Autodesk Fusion 360 part; units mm, degrees
(part 2 of 6)
  line L897 (212.8261, -84.2499) -> (212.026, -84.2499)
  line L898 (212.026, -84.2499) -> (212.026, -78.3011)
  line L899 (212.026, -78.3011) -> (212.8261, -78.3011)
  line L900 (212.8261, -78.3011) -> (212.8261, -75.3509)
  line L901 (212.8261, -75.3509) -> (212.026, -75.3509)
  line L902 (212.026, -75.3509) -> (212.026, -74.3511)
  line L903 (212.026, -74.3511) -> (198.1761, -74.3511)
  line L904 (217.2261, -74.3511) -> (217.2261, -75.3509)
  line L905 (217.2261, -75.3509) -> (216.426, -75.3509)
  line L906 (216.426, -75.3509) -> (216.426, -78.3011)
  line L907 (216.426, -78.3011) -> (217.2261, -78.3011)
  line L908 (217.2261, -78.3011) -> (217.2261, -84.2499)
  line L909 (217.2261, -84.2499) -> (216.426, -84.2499)
  line L910 (216.426, -84.2499) -> (216.426, -87.2001)
  line L911 (216.426, -87.2001) -> (217.2261, -87.2001)
  line L912 (217.2261, -87.2001) -> (217.2261, -88.1999)
  line L913 (217.2261, -88.1999) -> (231.076, -88.1999)
  line L914 (231.076, -88.1999) -> (231.076, -87.2001)
  line L915 (231.076, -87.2001) -> (231.8761, -87.2001)
  line L916 (231.8761, -87.2001) -> (231.8761, -84.2499)
  line L917 (231.8761, -84.2499) -> (231.076, -84.2499)
  line L918 (231.076, -84.2499) -> (231.076, -78.3011)
  line L919 (231.076, -78.3011) -> (231.8761, -78.3011)
  line L920 (231.8761, -78.3011) -> (231.8761, -75.3509)
  line L921 (231.8761, -75.3509) -> (231.076, -75.3509)
  line L922 (231.076, -75.3509) -> (231.076, -74.3511)
  line L923 (231.076, -74.3511) -> (217.2261, -74.3511)
  line L924 (236.2761, -74.3511) -> (236.2761, -75.3509)
  line L925 (236.2761, -75.3509) -> (235.476, -75.3509)
  line L926 (235.476, -75.3509) -> (235.476, -78.3011)
  line L927 (235.476, -78.3011) -> (236.2761, -78.3011)
  line L928 (236.2761, -78.3011) -> (236.2761, -84.2499)
  line L929 (236.2761, -84.2499) -> (235.476, -84.2499)
  line L930 (235.476, -84.2499) -> (235.476, -87.2001)
  line L931 (235.476, -87.2001) -> (236.2761, -87.2001)
  line L932 (236.2761, -87.2001) -> (236.2761, -88.1999)
  line L933 (236.2761, -88.1999) -> (250.126, -88.1999)
  line L934 (250.126, -88.1999) -> (250.126, -87.2001)
  line L935 (250.126, -87.2001) -> (250.9261, -87.2001)
  line L936 (250.9261, -87.2001) -> (250.9261, -84.2499)
  line L937 (250.9261, -84.2499) -> (250.126, -84.2499)
  line L938 (250.126, -84.2499) -> (250.126, -78.3011)
  line L939 (250.126, -78.3011) -> (250.9261, -78.3011)
  line L940 (250.9261, -78.3011) -> (250.9261, -75.3509)
  line L941 (250.9261, -75.3509) -> (250.126, -75.3509)
  line L942 (250.126, -75.3509) -> (250.126, -74.3511)
  line L943 (250.126, -74.3511) -> (236.2761, -74.3511)
  line L944 (307.7131, -74.3511) -> (307.7131, -75.3509)
  line L945 (307.7131, -75.3509) -> (306.914, -75.3509)
  line L946 (306.914, -75.3509) -> (306.914, -78.3011)
  line L947 (306.914, -78.3011) -> (307.7131, -78.3011)
  line L948 (307.7131, -78.3011) -> (307.7131, -84.2499)
  line L949 (307.7131, -84.2499) -> (306.914, -84.2499)
  line L950 (306.914, -84.2499) -> (306.914, -87.2001)
  line L951 (306.914, -87.2001) -> (307.7131, -87.2001)
  line L952 (307.7131, -87.2001) -> (307.7131, -88.1999)
  line L953 (307.7131, -88.1999) -> (321.564, -88.1999)
  line L954 (321.564, -88.1999) -> (321.564, -87.2001)
  line L955 (321.564, -87.2001) -> (322.363, -87.2001)
  line L956 (322.363, -87.2001) -> (322.363, -84.2499)
  line L957 (322.363, -84.2499) -> (321.564, -84.2499)
  line L958 (321.564, -84.2499) -> (321.564, -78.3011)
  line L959 (321.564, -78.3011) -> (322.363, -78.3011)
  line L960 (322.363, -78.3011) -> (322.363, -75.3509)
  line L961 (322.363, -75.3509) -> (321.564, -75.3509)
  line L962 (321.564, -75.3509) -> (321.564, -74.3511)
  line L963 (321.564, -74.3511) -> (307.7131, -74.3511)
  line L964 (17.201, -55.3011) -> (17.201, -56.301)
  line L965 (17.201, -56.301) -> (16.401, -56.301)
  line L966 (16.401, -56.301) -> (16.401, -59.25)
  line L967 (16.401, -59.25) -> (17.201, -59.25)
  line L968 (17.201, -59.25) -> (17.201, -65.1999)
  line L969 (17.201, -65.1999) -> (16.401, -65.1999)
  line L970 (16.401, -65.1999) -> (16.401, -68.1501)
  line L971 (16.401, -68.1501) -> (17.201, -68.1501)
  line L972 (17.201, -68.1501) -> (17.201, -69.1499)
  line L973 (17.201, -69.1499) -> (31.051, -69.1499)
  line L974 (31.051, -69.1499) -> (31.051, -68.1501)
  line L975 (31.051, -68.1501) -> (31.8511, -68.1501)
  line L976 (31.8511, -68.1501) -> (31.8511, -65.1999)
  line L977 (31.8511, -65.1999) -> (31.051, -65.1999)
  line L978 (31.051, -65.1999) -> (31.051, -59.25)
  line L979 (31.051, -59.25) -> (31.8511, -59.25)
  line L980 (31.8511, -59.25) -> (31.8511, -56.301)
  line L981 (31.8511, -56.301) -> (31.051, -56.301)
  line L982 (31.051, -56.301) -> (31.051, -55.3011)
  line L983 (31.051, -55.3011) -> (17.201, -55.3011)
  line L984 (41.0131, -55.3011) -> (41.0131, -56.301)
  line L985 (41.0131, -56.301) -> (40.213, -56.301)
  line L986 (40.213, -56.301) -> (40.213, -59.25)
  line L987 (40.213, -59.25) -> (41.0131, -59.25)
  line L988 (41.0131, -59.25) -> (41.0131, -65.1999)
  line L989 (41.0131, -65.1999) -> (40.213, -65.1999)
  line L990 (40.213, -65.1999) -> (40.213, -68.1501)
  line L991 (40.213, -68.1501) -> (41.0131, -68.1501)
  line L992 (41.0131, -68.1501) -> (41.0131, -69.1499)
  line L993 (41.0131, -69.1499) -> (54.8629, -69.1499)
  line L994 (54.8629, -69.1499) -> (54.8629, -68.1501)
  line L995 (54.8629, -68.1501) -> (55.663, -68.1501)
  line L996 (55.663, -68.1501) -> (55.663, -65.1999)
  line L997 (55.663, -65.1999) -> (54.8629, -65.1999)
  line L998 (54.8629, -65.1999) -> (54.8629, -59.25)
  line L999 (54.8629, -59.25) -> (55.663, -59.25)
  line L1000 (55.663, -59.25) -> (55.663, -56.301)
  line L1001 (55.663, -56.301) -> (54.8629, -56.301)
  line L1002 (54.8629, -56.301) -> (54.8629, -55.3011)
  line L1003 (54.8629, -55.3011) -> (41.0131, -55.3011)
  line L1004 (60.0631, -55.3011) -> (60.0631, -56.301)
  line L1005 (60.0631, -56.301) -> (59.263, -56.301)
  line L1006 (59.263, -56.301) -> (59.263, -59.25)
  line L1007 (59.263, -59.25) -> (60.0631, -59.25)
  line L1008 (60.0631, -59.25) -> (60.0631, -65.1999)
  line L1009 (60.0631, -65.1999) -> (59.263, -65.1999)
  line L1010 (59.263, -65.1999) -> (59.263, -68.1501)
  line L1011 (59.263, -68.1501) -> (60.0631, -68.1501)
  line L1012 (60.0631, -68.1501) -> (60.0631, -69.1499)
  line L1013 (60.0631, -69.1499) -> (73.9129, -69.1499)
  line L1014 (73.9129, -69.1499) -> (73.9129, -68.1501)
  line L1015 (73.9129, -68.1501) -> (74.713, -68.1501)
  line L1016 (74.713, -68.1501) -> (74.713, -65.1999)
  line L1017 (74.713, -65.1999) -> (73.9129, -65.1999)
  line L1018 (73.9129, -65.1999) -> (73.9129, -59.25)
  line L1019 (73.9129, -59.25) -> (74.713, -59.25)
  line L1020 (74.713, -59.25) -> (74.713, -56.301)
  line L1021 (74.713, -56.301) -> (73.9129, -56.301)
  line L1022 (73.9129, -56.301) -> (73.9129, -55.3011)
  line L1023 (73.9129, -55.3011) -> (60.0631, -55.3011)
  line L1024 (79.1131, -55.3011) -> (79.1131, -56.301)
  line L1025 (79.1131, -56.301) -> (78.313, -56.301)
  line L1026 (78.313, -56.301) -> (78.313, -59.25)
  line L1027 (78.313, -59.25) -> (79.1131, -59.25)
  line L1028 (79.1131, -59.25) -> (79.1131, -65.1999)
  line L1029 (79.1131, -65.1999) -> (78.313, -65.1999)
  line L1030 (78.313, -65.1999) -> (78.313, -68.1501)
  line L1031 (78.313, -68.1501) -> (79.1131, -68.1501)
  line L1032 (79.1131, -68.1501) -> (79.1131, -69.1499)
  line L1033 (79.1131, -69.1499) -> (92.9629, -69.1499)
  line L1034 (92.9629, -69.1499) -> (92.9629, -68.1501)
  line L1035 (92.9629, -68.1501) -> (93.763, -68.1501)
  line L1036 (93.763, -68.1501) -> (93.763, -65.1999)
  line L1037 (93.763, -65.1999) -> (92.9629, -65.1999)
  line L1038 (92.9629, -65.1999) -> (92.9629, -59.25)
  line L1039 (92.9629, -59.25) -> (93.763, -59.25)
  line L1040 (93.763, -59.25) -> (93.763, -56.301)
  line L1041 (93.763, -56.301) -> (92.9629, -56.301)
  line L1042 (92.9629, -56.301) -> (92.9629, -55.3011)
  line L1043 (92.9629, -55.3011) -> (79.1131, -55.3011)
  line L1044 (98.1631, -55.3011) -> (98.1631, -56.301)
  line L1045 (98.1631, -56.301) -> (97.363, -56.301)
  line L1046 (97.363, -56.301) -> (97.363, -59.25)
  line L1047 (97.363, -59.25) -> (98.1631, -59.25)
  line L1048 (98.1631, -59.25) -> (98.1631, -65.1999)
  line L1049 (98.1631, -65.1999) -> (97.363, -65.1999)
  line L1050 (97.363, -65.1999) -> (97.363, -68.1501)
  line L1051 (97.363, -68.1501) -> (98.1631, -68.1501)
  line L1052 (98.1631, -68.1501) -> (98.1631, -69.1499)
  line L1053 (98.1631, -69.1499) -> (112.0129, -69.1499)
  line L1054 (112.0129, -69.1499) -> (112.0129, -68.1501)
  line L1055 (112.0129, -68.1501) -> (112.813, -68.1501)
  line L1056 (112.813, -68.1501) -> (112.813, -65.1999)
  line L1057 (112.813, -65.1999) -> (112.0129, -65.1999)
  line L1058 (112.0129, -65.1999) -> (112.0129, -59.25)
  line L1059 (112.0129, -59.25) -> (112.813, -59.25)
  line L1060 (112.813, -59.25) -> (112.813, -56.301)
  line L1061 (112.813, -56.301) -> (112.0129, -56.301)
  line L1062 (112.0129, -56.301) -> (112.0129, -55.3011)
  line L1063 (112.0129, -55.3011) -> (98.1631, -55.3011)
  line L1064 (117.2131, -55.3011) -> (117.2131, -56.301)
  line L1065 (117.2131, -56.301) -> (116.413, -56.301)
  line L1066 (116.413, -56.301) -> (116.413, -59.25)
  line L1067 (116.413, -59.25) -> (117.2131, -59.25)
  line L1068 (117.2131, -59.25) -> (117.2131, -65.1999)
  line L1069 (117.2131, -65.1999) -> (116.413, -65.1999)
  line L1070 (116.413, -65.1999) -> (116.413, -68.1501)
  line L1071 (116.413, -68.1501) -> (117.2131, -68.1501)
  line L1072 (117.2131, -68.1501) -> (117.2131, -69.1499)
  line L1073 (117.2131, -69.1499) -> (131.0629, -69.1499)
  line L1074 (131.0629, -69.1499) -> (131.0629, -68.1501)
  line L1075 (131.0629, -68.1501) -> (131.863, -68.1501)
  line L1076 (131.863, -68.1501) -> (131.863, -65.1999)
  line L1077 (131.863, -65.1999) -> (131.0629, -65.1999)
  line L1078 (131.0629, -65.1999) -> (131.0629, -59.25)
  line L1079 (131.0629, -59.25) -> (131.863, -59.25)
  line L1080 (131.863, -59.25) -> (131.863, -56.301)
  line L1081 (131.863, -56.301) -> (131.0629, -56.301)
  line L1082 (131.0629, -56.301) -> (131.0629, -55.3011)
  line L1083 (131.0629, -55.3011) -> (117.2131, -55.3011)
  line L1084 (136.2631, -55.3011) -> (136.2631, -56.301)
  line L1085 (136.2631, -56.301) -> (135.463, -56.301)
  line L1086 (135.463, -56.301) -> (135.463, -59.25)
  line L1087 (135.463, -59.25) -> (136.2631, -59.25)
  line L1088 (136.2631, -59.25) -> (136.2631, -65.1999)
  line L1089 (136.2631, -65.1999) -> (135.463, -65.1999)
  line L1090 (135.463, -65.1999) -> (135.463, -68.1501)
  line L1091 (135.463, -68.1501) -> (136.2631, -68.1501)
  line L1092 (136.2631, -68.1501) -> (136.2631, -69.1499)
  line L1093 (136.2631, -69.1499) -> (150.1129, -69.1499)
  line L1094 (150.1129, -69.1499) -> (150.1129, -68.1501)
  line L1095 (150.1129, -68.1501) -> (150.913, -68.1501)
  line L1096 (150.913, -68.1501) -> (150.913, -65.1999)
  line L1097 (150.913, -65.1999) -> (150.1129, -65.1999)
  line L1098 (150.1129, -65.1999) -> (150.1129, -59.25)
  line L1099 (150.1129, -59.25) -> (150.913, -59.25)
  line L1100 (150.913, -59.25) -> (150.913, -56.301)
  line L1101 (150.913, -56.301) -> (150.1129, -56.301)
  line L1102 (150.1129, -56.301) -> (150.1129, -55.3011)
  line L1103 (150.1129, -55.3011) -> (136.2631, -55.3011)
  line L1104 (155.3131, -55.3011) -> (155.3131, -56.301)
  line L1105 (155.3131, -56.301) -> (154.513, -56.301)
  line L1106 (154.513, -56.301) -> (154.513, -59.25)
  line L1107 (154.513, -59.25) -> (155.3131, -59.25)
  line L1108 (155.3131, -59.25) -> (155.3131, -65.1999)
  line L1109 (155.3131, -65.1999) -> (154.513, -65.1999)
  line L1110 (154.513, -65.1999) -> (154.513, -68.1501)
  line L1111 (154.513, -68.1501) -> (155.3131, -68.1501)
  line L1112 (155.3131, -68.1501) -> (155.3131, -69.1499)
  line L1113 (155.3131, -69.1499) -> (169.1629, -69.1499)
  line L1114 (169.1629, -69.1499) -> (169.1629, -68.1501)
  line L1115 (169.1629, -68.1501) -> (169.963, -68.1501)
  line L1116 (169.963, -68.1501) -> (169.963, -65.1999)
  line L1117 (169.963, -65.1999) -> (169.1629, -65.1999)
  line L1118 (169.1629, -65.1999) -> (169.1629, -59.25)
  line L1119 (169.1629, -59.25) -> (169.963, -59.25)
  line L1120 (169.963, -59.25) -> (169.963, -56.301)
  line L1121 (169.963, -56.301) -> (169.1629, -56.301)
  line L1122 (169.1629, -56.301) -> (169.1629, -55.3011)
  line L1123 (169.1629, -55.3011) -> (155.3131, -55.3011)
  line L1124 (174.3631, -55.3011) -> (174.3631, -56.301)
  line L1125 (174.3631, -56.301) -> (173.563, -56.301)
  line L1126 (173.563, -56.301) -> (173.563, -59.25)
  line L1127 (173.563, -59.25) -> (174.3631, -59.25)
  line L1128 (174.3631, -59.25) -> (174.3631, -65.1999)
  line L1129 (174.3631, -65.1999) -> (173.563, -65.1999)
  line L1130 (173.563, -65.1999) -> (173.563, -68.1501)
  line L1131 (173.563, -68.1501) -> (174.3631, -68.1501)
  line L1132 (174.3631, -68.1501) -> (174.3631, -69.1499)
  line L1133 (174.3631, -69.1499) -> (188.2129, -69.1499)
  line L1134 (188.2129, -69.1499) -> (188.2129, -68.1501)
  line L1135 (188.2129, -68.1501) -> (189.013, -68.1501)
  line L1136 (189.013, -68.1501) -> (189.013, -65.1999)
  line L1137 (189.013, -65.1999) -> (188.2129, -65.1999)
  line L1138 (188.2129, -65.1999) -> (188.2129, -59.25)
  line L1139 (188.2129, -59.25) -> (189.013, -59.25)
  line L1140 (189.013, -59.25) -> (189.013, -56.301)
  line L1141 (189.013, -56.301) -> (188.2129, -56.301)
  line L1142 (188.2129, -56.301) -> (188.2129, -55.3011)
  line L1143 (188.2129, -55.3011) -> (174.3631, -55.3011)
  line L1144 (193.4131, -55.3011) -> (193.4131, -56.301)
  line L1145 (193.4131, -56.301) -> (192.613, -56.301)
  line L1146 (192.613, -56.301) -> (192.613, -59.25)
  line L1147 (192.613, -59.25) -> (193.4131, -59.25)
  line L1148 (193.4131, -59.25) -> (193.4131, -65.1999)
  line L1149 (193.4131, -65.1999) -> (192.613, -65.1999)
  line L1150 (192.613, -65.1999) -> (192.613, -68.1501)
  line L1151 (192.613, -68.1501) -> (193.4131, -68.1501)
  line L1152 (193.4131, -68.1501) -> (193.4131, -69.1499)
  line L1153 (193.4131, -69.1499) -> (207.2629, -69.1499)
  line L1154 (207.2629, -69.1499) -> (207.2629, -68.1501)
  line L1155 (207.2629, -68.1501) -> (208.063, -68.1501)
  line L1156 (208.063, -68.1501) -> (208.063, -65.1999)
  line L1157 (208.063, -65.1999) -> (207.2629, -65.1999)
  line L1158 (207.2629, -65.1999) -> (207.2629, -59.25)
  line L1159 (207.2629, -59.25) -> (208.063, -59.25)
  line L1160 (208.063, -59.25) -> (208.063, -56.301)
  line L1161 (208.063, -56.301) -> (207.2629, -56.301)
  line L1162 (207.2629, -56.301) -> (207.2629, -55.3011)
  line L1163 (207.2629, -55.3011) -> (193.4131, -55.3011)
  line L1164 (212.4631, -55.3011) -> (212.4631, -56.301)
  line L1165 (212.4631, -56.301) -> (211.663, -56.301)
  line L1166 (211.663, -56.301) -> (211.663, -59.25)
  line L1167 (211.663, -59.25) -> (212.4631, -59.25)
  line L1168 (212.4631, -59.25) -> (212.4631, -65.1999)
  line L1169 (212.4631, -65.1999) -> (211.663, -65.1999)
  line L1170 (211.663, -65.1999) -> (211.663, -68.1501)
  line L1171 (211.663, -68.1501) -> (212.4631, -68.1501)
  line L1172 (212.4631, -68.1501) -> (212.4631, -69.1499)
  line L1173 (212.4631, -69.1499) -> (226.3129, -69.1499)
  line L1174 (226.3129, -69.1499) -> (226.3129, -68.1501)
  line L1175 (226.3129, -68.1501) -> (227.113, -68.1501)
  line L1176 (227.113, -68.1501) -> (227.113, -65.1999)
  line L1177 (227.113, -65.1999) -> (226.3129, -65.1999)
  line L1178 (226.3129, -65.1999) -> (226.3129, -59.25)
  line L1179 (226.3129, -59.25) -> (227.113, -59.25)
  line L1180 (227.113, -59.25) -> (227.113, -56.301)
  line L1181 (227.113, -56.301) -> (226.3129, -56.301)
  line L1182 (226.3129, -56.301) -> (226.3129, -55.3011)
  line L1183 (226.3129, -55.3011) -> (212.4631, -55.3011)
  line L1184 (231.5131, -55.3011) -> (231.5131, -56.301)
  line L1185 (231.5131, -56.301) -> (230.713, -56.301)
  line L1186 (230.713, -56.301) -> (230.713, -59.25)
  line L1187 (230.713, -59.25) -> (231.5131, -59.25)
  line L1188 (231.5131, -59.25) -> (231.5131, -65.1999)
  line L1189 (231.5131, -65.1999) -> (230.713, -65.1999)
  line L1190 (230.713, -65.1999) -> (230.713, -68.1501)
  line L1191 (230.713, -68.1501) -> (231.5131, -68.1501)
  line L1192 (231.5131, -68.1501) -> (231.5131, -69.1499)
  line L1193 (231.5131, -69.1499) -> (245.3629, -69.1499)
  line L1194 (245.3629, -69.1499) -> (245.3629, -68.1501)
  line L1195 (245.3629, -68.1501) -> (246.163, -68.1501)
  line L1196 (246.163, -68.1501) -> (246.163, -65.1999)
  line L1197 (246.163, -65.1999) -> (245.3629, -65.1999)
  line L1198 (245.3629, -65.1999) -> (245.3629, -59.25)
  line L1199 (245.3629, -59.25) -> (246.163, -59.25)
  line L1200 (246.163, -59.25) -> (246.163, -56.301)
  line L1201 (246.163, -56.301) -> (245.3629, -56.301)
  line L1202 (245.3629, -56.301) -> (245.3629, -55.3011)
  line L1203 (245.3629, -55.3011) -> (231.5131, -55.3011)
  line L1204 (250.5631, -55.3011) -> (250.5631, -56.301)
  line L1205 (250.5631, -56.301) -> (249.763, -56.301)
  line L1206 (249.763, -56.301) -> (249.763, -59.25)
  line L1207 (249.763, -59.25) -> (250.5631, -59.25)
  line L1208 (250.5631, -59.25) -> (250.5631, -65.1999)
  line L1209 (250.5631, -65.1999) -> (249.763, -65.1999)
  line L1210 (249.763, -65.1999) -> (249.763, -68.1501)
  line L1211 (249.763, -68.1501) -> (250.5631, -68.1501)
  line L1212 (250.5631, -68.1501) -> (250.5631, -69.1499)
  line L1213 (250.5631, -69.1499) -> (264.4129, -69.1499)
  line L1214 (264.4129, -69.1499) -> (264.4129, -68.1501)
  line L1215 (264.4129, -68.1501) -> (265.213, -68.1501)
  line L1216 (265.213, -68.1501) -> (265.213, -65.1999)
  line L1217 (265.213, -65.1999) -> (264.4129, -65.1999)
  line L1218 (264.4129, -65.1999) -> (264.4129, -59.25)
  line L1219 (264.4129, -59.25) -> (265.213, -59.25)
  line L1220 (265.213, -59.25) -> (265.213, -56.301)
  line L1221 (265.213, -56.301) -> (264.4129, -56.301)
  line L1222 (264.4129, -56.301) -> (264.4129, -55.3011)
  line L1223 (264.4129, -55.3011) -> (250.5631, -55.3011)
  line L1224 (274.3756, -55.3011) -> (274.3756, -56.301)
  line L1225 (274.3756, -56.301) -> (273.5765, -56.301)
  line L1226 (273.5765, -56.301) -> (273.5765, -59.25)
  line L1227 (273.5765, -59.25) -> (274.3756, -59.25)
  line L1228 (274.3756, -59.25) -> (274.3756, -65.1999)
  line L1229 (274.3756, -65.1999) -> (273.5765, -65.1999)
  line L1230 (273.5765, -65.1999) -> (273.5765, -68.1501)
  line L1231 (273.5765, -68.1501) -> (274.3756, -68.1501)
  line L1232 (274.3756, -68.1501) -> (274.3756, -69.1499)
  line L1233 (274.3756, -69.1499) -> (288.2265, -69.1499)
  line L1234 (288.2265, -69.1499) -> (288.2265, -68.1501)
  line L1235 (288.2265, -68.1501) -> (289.0255, -68.1501)
  line L1236 (289.0255, -68.1501) -> (289.0255, -65.1999)
  line L1237 (289.0255, -65.1999) -> (288.2265, -65.1999)
  line L1238 (288.2265, -65.1999) -> (288.2265, -59.25)
  line L1239 (288.2265, -59.25) -> (289.0255, -59.25)
  line L1240 (289.0255, -59.25) -> (289.0255, -56.301)
  line L1241 (289.0255, -56.301) -> (288.2265, -56.301)
  line L1242 (288.2265, -56.301) -> (288.2265, -55.3011)
  line L1243 (288.2265, -55.3011) -> (274.3756, -55.3011)
  line L1244 (307.7131, -55.3011) -> (307.7131, -56.301)
  line L1245 (307.7131, -56.301) -> (306.914, -56.301)
  line L1246 (306.914, -56.301) -> (306.914, -59.25)
  line L1247 (306.914, -59.25) -> (307.7131, -59.25)
  line L1248 (307.7131, -59.25) -> (307.7131, -65.1999)
  line L1249 (307.7131, -65.1999) -> (306.914, -65.1999)
  line L1250 (306.914, -65.1999) -> (306.914, -68.1501)
  line L1251 (306.914, -68.1501) -> (307.7131, -68.1501)
  line L1252 (307.7131, -68.1501) -> (307.7131, -69.1499)
  line L1253 (307.7131, -69.1499) -> (321.564, -69.1499)
  line L1254 (321.564, -69.1499) -> (321.564, -68.1501)
  line L1255 (321.564, -68.1501) -> (322.363, -68.1501)
  line L1256 (322.363, -68.1501) -> (322.363, -65.1999)
  line L1257 (322.363, -65.1999) -> (321.564, -65.1999)
  line L1258 (321.564, -65.1999) -> (321.564, -59.25)
  line L1259 (321.564, -59.25) -> (322.363, -59.25)
  line L1260 (322.363, -59.25) -> (322.363, -56.301)
  line L1261 (322.363, -56.301) -> (321.564, -56.301)
  line L1262 (321.564, -56.301) -> (321.564, -55.3011)
  line L1263 (321.564, -55.3011) -> (307.7131, -55.3011)
  line L1264 (269.6131, -36.2511) -> (269.6131, -37.251)
  line L1265 (269.6131, -37.251) -> (268.814, -37.251)
  line L1266 (268.814, -37.251) -> (268.814, -40.2)
  line L1267 (268.814, -40.2) -> (269.6131, -40.2)
  line L1268 (269.6131, -40.2) -> (269.6131, -40.9501)
  line L1269 (269.6131, -40.9501) -> (267.9382, -40.9501)
  line L1270 (267.9382, -40.9501) -> (267.9382, -37.7211)
  line L1271 (267.9382, -37.7211) -> (266.2132, -37.7211)
  line L1272 (266.2132, -37.7211) -> (266.2132, -36.8009)
  line L1273 (266.2132, -36.8009) -> (263.063, -36.8009)
  line L1274 (263.063, -36.8009) -> (263.063, -37.7211)
  line L1275 (263.063, -37.7211) -> (261.338, -37.7211)
  line L1276 (261.338, -37.7211) -> (261.338, -40.9501)
  line L1277 (261.338, -40.9501) -> (260.513, -40.9501)
  line L1278 (260.513, -40.9501) -> (260.513, -43.5999)
  line L1279 (260.513, -43.5999) -> (261.338, -43.5999)
  line L1280 (261.338, -43.5999) -> (261.338, -49.871)
  line L1281 (261.338, -49.871) -> (263.063, -49.871)
  line L1282 (263.063, -49.871) -> (263.063, -50.85)
  line L1283 (263.063, -50.85) -> (266.2132, -50.85)
  line L1284 (266.2132, -50.85) -> (266.2132, -49.871)
  line L1285 (266.2132, -49.871) -> (267.9382, -49.871)
  line L1286 (267.9382, -49.871) -> (267.9382, -45.4009)
  line L1287 (267.9382, -45.4009) -> (269.6131, -45.4009)
  line L1288 (269.6131, -45.4009) -> (269.6131, -46.151)
  line L1289 (269.6131, -46.151) -> (268.814, -46.151)
  line L1290 (268.814, -46.151) -> (268.814, -49.1001)
  line L1291 (268.814, -49.1001) -> (269.6131, -49.1001)
  line L1292 (269.6131, -49.1001) -> (269.6131, -50.0999)
  line L1293 (269.6131, -50.0999) -> (283.464, -50.0999)
  line L1294 (283.464, -50.0999) -> (283.464, -49.1001)
  line L1295 (283.464, -49.1001) -> (284.263, -49.1001)
  line L1296 (284.263, -49.1001) -> (284.263, -46.151)
  line L1297 (284.263, -46.151) -> (283.464, -46.151)
  line L1298 (283.464, -46.151) -> (283.464, -45.4009)
  line L1299 (283.464, -45.4009) -> (285.1388, -45.4009)
  line L1300 (285.1388, -45.4009) -> (285.1388, -49.871)
  line L1301 (285.1388, -49.871) -> (286.8639, -49.871)
  line L1302 (286.8639, -49.871) -> (286.8639, -50.85)
  line L1303 (286.8639, -50.85) -> (290.0124, -50.85)
  line L1304 (290.0124, -50.85) -> (290.0124, -49.871)
  line L1305 (290.0124, -49.871) -> (291.7375, -49.871)
  line L1306 (291.7375, -49.871) -> (291.7375, -43.5999)
  line L1307 (291.7375, -43.5999) -> (292.563, -43.5999)
  line L1308 (292.563, -43.5999) -> (292.563, -40.9501)
  line L1309 (292.563, -40.9501) -> (291.7375, -40.9501)
  line L1310 (291.7375, -40.9501) -> (291.7375, -37.7211)
  line L1311 (291.7375, -37.7211) -> (290.0124, -37.7211)
  line L1312 (290.0124, -37.7211) -> (290.0124, -36.8009)
  line L1313 (290.0124, -36.8009) -> (286.8639, -36.8009)
  line L1314 (286.8639, -36.8009) -> (286.8639, -37.7211)
  line L1315 (286.8639, -37.7211) -> (285.1388, -37.7211)
  line L1316 (285.1388, -37.7211) -> (285.1388, -40.9501)
  line L1317 (285.1388, -40.9501) -> (283.464, -40.9501)
  line L1318 (283.464, -40.9501) -> (283.464, -40.2)
  line L1319 (283.464, -40.2) -> (284.263, -40.2)
  line L1320 (284.263, -40.2) -> (284.263, -37.251)
  line L1321 (284.263, -37.251) -> (283.464, -37.251)
  line L1322 (283.464, -37.251) -> (283.464, -36.2511)
  line L1323 (283.464, -36.2511) -> (269.6131, -36.2511)
  line L1324 (12.438, -36.2511) -> (12.438, -37.251)
  line L1325 (12.438, -37.251) -> (11.638, -37.251)
  line L1326 (11.638, -37.251) -> (11.638, -40.2)
  line L1327 (11.638, -40.2) -> (12.438, -40.2)
  line L1328 (12.438, -40.2) -> (12.438, -46.151)
  line L1329 (12.438, -46.151) -> (11.638, -46.151)
  line L1330 (11.638, -46.151) -> (11.638, -49.1001)
  line L1331 (11.638, -49.1001) -> (12.438, -49.1001)
  line L1332 (12.438, -49.1001) -> (12.438, -50.0999)
  line L1333 (12.438, -50.0999) -> (26.288, -50.0999)
  line L1334 (26.288, -50.0999) -> (26.288, -49.1001)
  line L1335 (26.288, -49.1001) -> (27.088, -49.1001)
  line L1336 (27.088, -49.1001) -> (27.088, -46.151)
  line L1337 (27.088, -46.151) -> (26.288, -46.151)
  line L1338 (26.288, -46.151) -> (26.288, -40.2)
  line L1339 (26.288, -40.2) -> (27.088, -40.2)
  line L1340 (27.088, -40.2) -> (27.088, -37.251)
  line L1341 (27.088, -37.251) -> (26.288, -37.251)
  line L1342 (26.288, -37.251) -> (26.288, -36.2511)
  line L1343 (26.288, -36.2511) -> (12.438, -36.2511)
  line L1344 (31.4881, -36.2511) -> (31.4881, -37.251)
  line L1345 (31.4881, -37.251) -> (30.688, -37.251)
  line L1346 (30.688, -37.251) -> (30.688, -40.2)
  line L1347 (30.688, -40.2) -> (31.4881, -40.2)
  line L1348 (31.4881, -40.2) -> (31.4881, -46.151)
  line L1349 (31.4881, -46.151) -> (30.688, -46.151)
  line L1350 (30.688, -46.151) -> (30.688, -49.1001)
  line L1351 (30.688, -49.1001) -> (31.4881, -49.1001)
  line L1352 (31.4881, -49.1001) -> (31.4881, -50.0999)
  line L1353 (31.4881, -50.0999) -> (45.3379, -50.0999)
  line L1354 (45.3379, -50.0999) -> (45.3379, -49.1001)
  line L1355 (45.3379, -49.1001) -> (46.138, -49.1001)
  line L1356 (46.138, -49.1001) -> (46.138, -46.151)
  line L1357 (46.138, -46.151) -> (45.3379, -46.151)
  line L1358 (45.3379, -46.151) -> (45.3379, -40.2)
  line L1359 (45.3379, -40.2) -> (46.138, -40.2)
  line L1360 (46.138, -40.2) -> (46.138, -37.251)
  line L1361 (46.138, -37.251) -> (45.3379, -37.251)
  line L1362 (45.3379, -37.251) -> (45.3379, -36.2511)
  line L1363 (45.3379, -36.2511) -> (31.4881, -36.2511)
  line L1364 (50.5381, -36.2511) -> (50.5381, -37.251)
  line L1365 (50.5381, -37.251) -> (49.738, -37.251)
  line L1366 (49.738, -37.251) -> (49.738, -40.2)
  line L1367 (49.738, -40.2) -> (50.5381, -40.2)
  line L1368 (50.5381, -40.2) -> (50.5381, -46.151)
  line L1369 (50.5381, -46.151) -> (49.738, -46.151)
  line L1370 (49.738, -46.151) -> (49.738, -49.1001)
  line L1371 (49.738, -49.1001) -> (50.5381, -49.1001)
  line L1372 (50.5381, -49.1001) -> (50.5381, -50.0999)
  line L1373 (50.5381, -50.0999) -> (64.3879, -50.0999)
  line L1374 (64.3879, -50.0999) -> (64.3879, -49.1001)
  line L1375 (64.3879, -49.1001) -> (65.188, -49.1001)
  line L1376 (65.188, -49.1001) -> (65.188, -46.151)
  line L1377 (65.188, -46.151) -> (64.3879, -46.151)
  line L1378 (64.3879, -46.151) -> (64.3879, -40.2)
  line L1379 (64.3879, -40.2) -> (65.188, -40.2)
  line L1380 (65.188, -40.2) -> (65.188, -37.251)
  line L1381 (65.188, -37.251) -> (64.3879, -37.251)
  line L1382 (64.3879, -37.251) -> (64.3879, -36.2511)
  line L1383 (64.3879, -36.2511) -> (50.5381, -36.2511)
  line L1384 (69.5881, -36.2511) -> (69.5881, -37.251)
  line L1385 (69.5881, -37.251) -> (68.788, -37.251)
  line L1386 (68.788, -37.251) -> (68.788, -40.2)
  line L1387 (68.788, -40.2) -> (69.5881, -40.2)
  line L1388 (69.5881, -40.2) -> (69.5881, -46.151)
  line L1389 (69.5881, -46.151) -> (68.788, -46.151)
  line L1390 (68.788, -46.151) -> (68.788, -49.1001)
  line L1391 (68.788, -49.1001) -> (69.5881, -49.1001)
  line L1392 (69.5881, -49.1001) -> (69.5881, -50.0999)
  line L1393 (69.5881, -50.0999) -> (83.4379, -50.0999)
  line L1394 (83.4379, -50.0999) -> (83.4379, -49.1001)
  line L1395 (83.4379, -49.1001) -> (84.238, -49.1001)
  line L1396 (84.238, -49.1001) -> (84.238, -46.151)
  line L1397 (84.238, -46.151) -> (83.4379, -46.151)
  line L1398 (83.4379, -46.151) -> (83.4379, -40.2)
  line L1399 (83.4379, -40.2) -> (84.238, -40.2)
  line L1400 (84.238, -40.2) -> (84.238, -37.251)
  line L1401 (84.238, -37.251) -> (83.4379, -37.251)
  line L1402 (83.4379, -37.251) -> (83.4379, -36.2511)
  line L1403 (83.4379, -36.2511) -> (69.5881, -36.2511)
  line L1404 (88.6381, -36.2511) -> (88.6381, -37.251)
  line L1405 (88.6381, -37.251) -> (87.838, -37.251)
  line L1406 (87.838, -37.251) -> (87.838, -40.2)
  line L1407 (87.838, -40.2) -> (88.6381, -40.2)
  line L1408 (88.6381, -40.2) -> (88.6381, -46.151)
  line L1409 (88.6381, -46.151) -> (87.838, -46.151)
  line L1410 (87.838, -46.151) -> (87.838, -49.1001)
  line L1411 (87.838, -49.1001) -> (88.6381, -49.1001)
  line L1412 (88.6381, -49.1001) -> (88.6381, -50.0999)
  line L1413 (88.6381, -50.0999) -> (102.4879, -50.0999)
  line L1414 (102.4879, -50.0999) -> (102.4879, -49.1001)
  line L1415 (102.4879, -49.1001) -> (103.288, -49.1001)
  line L1416 (103.288, -49.1001) -> (103.288, -46.151)
  line L1417 (103.288, -46.151) -> (102.4879, -46.151)
  line L1418 (102.4879, -46.151) -> (102.4879, -40.2)
  line L1419 (102.4879, -40.2) -> (103.288, -40.2)
  line L1420 (103.288, -40.2) -> (103.288, -37.251)
  line L1421 (103.288, -37.251) -> (102.4879, -37.251)
  line L1422 (102.4879, -37.251) -> (102.4879, -36.2511)
  line L1423 (102.4879, -36.2511) -> (88.6381, -36.2511)
  line L1424 (107.6881, -36.2511) -> (107.6881, -37.251)
  line L1425 (107.6881, -37.251) -> (106.888, -37.251)
  line L1426 (106.888, -37.251) -> (106.888, -40.2)
  line L1427 (106.888, -40.2) -> (107.6881, -40.2)
  line L1428 (107.6881, -40.2) -> (107.6881, -46.151)
  line L1429 (107.6881, -46.151) -> (106.888, -46.151)
  line L1430 (106.888, -46.151) -> (106.888, -49.1001)
  line L1431 (106.888, -49.1001) -> (107.6881, -49.1001)
  line L1432 (107.6881, -49.1001) -> (107.6881, -50.0999)
  line L1433 (107.6881, -50.0999) -> (121.5379, -50.0999)
  line L1434 (121.5379, -50.0999) -> (121.5379, -49.1001)
  line L1435 (121.5379, -49.1001) -> (122.338, -49.1001)
  line L1436 (122.338, -49.1001) -> (122.338, -46.151)
  line L1437 (122.338, -46.151) -> (121.5379, -46.151)
  line L1438 (121.5379, -46.151) -> (121.5379, -40.2)
  line L1439 (121.5379, -40.2) -> (122.338, -40.2)
  line L1440 (122.338, -40.2) -> (122.338, -37.251)
  line L1441 (122.338, -37.251) -> (121.5379, -37.251)
  line L1442 (121.5379, -37.251) -> (121.5379, -36.2511)
  line L1443 (121.5379, -36.2511) -> (107.6881, -36.2511)
  line L1444 (126.7381, -36.2511) -> (126.7381, -37.251)
  line L1445 (126.7381, -37.251) -> (125.938, -37.251)
  line L1446 (125.938, -37.251) -> (125.938, -40.2)
  line L1447 (125.938, -40.2) -> (126.7381, -40.2)
  line L1448 (126.7381, -40.2) -> (126.7381, -46.151)
  line L1449 (126.7381, -46.151) -> (125.938, -46.151)
  line L1450 (125.938, -46.151) -> (125.938, -49.1001)
  line L1451 (125.938, -49.1001) -> (126.7381, -49.1001)
  line L1452 (126.7381, -49.1001) -> (126.7381, -50.0999)
  line L1453 (126.7381, -50.0999) -> (140.5879, -50.0999)
  line L1454 (140.5879, -50.0999) -> (140.5879, -49.1001)
  line L1455 (140.5879, -49.1001) -> (141.388, -49.1001)
  line L1456 (141.388, -49.1001) -> (141.388, -46.151)
  line L1457 (141.388, -46.151) -> (140.5879, -46.151)
  line L1458 (140.5879, -46.151) -> (140.5879, -40.2)
  line L1459 (140.5879, -40.2) -> (141.388, -40.2)
  line L1460 (141.388, -40.2) -> (141.388, -37.251)
  line L1461 (141.388, -37.251) -> (140.5879, -37.251)
  line L1462 (140.5879, -37.251) -> (140.5879, -36.2511)
  line L1463 (140.5879, -36.2511) -> (126.7381, -36.2511)
  line L1464 (145.7881, -36.2511) -> (145.7881, -37.251)
  line L1465 (145.7881, -37.251) -> (144.988, -37.251)
  line L1466 (144.988, -37.251) -> (144.988, -40.2)
  line L1467 (144.988, -40.2) -> (145.7881, -40.2)
  line L1468 (145.7881, -40.2) -> (145.7881, -46.151)
  line L1469 (145.7881, -46.151) -> (144.988, -46.151)
  line L1470 (144.988, -46.151) -> (144.988, -49.1001)
  line L1471 (144.988, -49.1001) -> (145.7881, -49.1001)
  line L1472 (145.7881, -49.1001) -> (145.7881, -50.0999)
  line L1473 (145.7881, -50.0999) -> (159.6379, -50.0999)
  line L1474 (159.6379, -50.0999) -> (159.6379, -49.1001)
  line L1475 (159.6379, -49.1001) -> (160.438, -49.1001)
  line L1476 (160.438, -49.1001) -> (160.438, -46.151)
  line L1477 (160.438, -46.151) -> (159.6379, -46.151)
  line L1478 (159.6379, -46.151) -> (159.6379, -40.2)
  line L1479 (159.6379, -40.2) -> (160.438, -40.2)
  line L1480 (160.438, -40.2) -> (160.438, -37.251)
  line L1481 (160.438, -37.251) -> (159.6379, -37.251)
  line L1482 (159.6379, -37.251) -> (159.6379, -36.2511)
  line L1483 (159.6379, -36.2511) -> (145.7881, -36.2511)
  line L1484 (164.8381, -36.2511) -> (164.8381, -37.251)
  line L1485 (164.8381, -37.251) -> (164.038, -37.251)
  line L1486 (164.038, -37.251) -> (164.038, -40.2)
  line L1487 (164.038, -40.2) -> (164.8381, -40.2)
  line L1488 (164.8381, -40.2) -> (164.8381, -46.151)
  line L1489 (164.8381, -46.151) -> (164.038, -46.151)
  line L1490 (164.038, -46.151) -> (164.038, -49.1001)
  line L1491 (164.038, -49.1001) -> (164.8381, -49.1001)
  line L1492 (164.8381, -49.1001) -> (164.8381, -50.0999)
  line L1493 (164.8381, -50.0999) -> (178.6879, -50.0999)
  line L1494 (178.6879, -50.0999) -> (178.6879, -49.1001)
  line L1495 (178.6879, -49.1001) -> (179.488, -49.1001)
  line L1496 (179.488, -49.1001) -> (179.488, -46.151)
  line L1497 (179.488, -46.151) -> (178.6879, -46.151)
  line L1498 (178.6879, -46.151) -> (178.6879, -40.2)
  line L1499 (178.6879, -40.2) -> (179.488, -40.2)
  line L1500 (179.488, -40.2) -> (179.488, -37.251)
  line L1501 (179.488, -37.251) -> (178.6879, -37.251)
  line L1502 (178.6879, -37.251) -> (178.6879, -36.2511)
  line L1503 (178.6879, -36.2511) -> (164.8381, -36.2511)
  line L1504 (183.8881, -36.2511) -> (183.8881, -37.251)
  line L1505 (183.8881, -37.251) -> (183.088, -37.251)
  line L1506 (183.088, -37.251) -> (183.088, -40.2)
  line L1507 (183.088, -40.2) -> (183.8881, -40.2)
  line L1508 (183.8881, -40.2) -> (183.8881, -46.151)
  line L1509 (183.8881, -46.151) -> (183.088, -46.151)
  line L1510 (183.088, -46.151) -> (183.088, -49.1001)
  line L1511 (183.088, -49.1001) -> (183.8881, -49.1001)
  line L1512 (183.8881, -49.1001) -> (183.8881, -50.0999)
  line L1513 (183.8881, -50.0999) -> (197.7379, -50.0999)
  line L1514 (197.7379, -50.0999) -> (197.7379, -49.1001)
  line L1515 (197.7379, -49.1001) -> (198.538, -49.1001)
  line L1516 (198.538, -49.1001) -> (198.538, -46.151)
  line L1517 (198.538, -46.151) -> (197.7379, -46.151)
  line L1518 (197.7379, -46.151) -> (197.7379, -40.2)
  line L1519 (197.7379, -40.2) -> (198.538, -40.2)
  line L1520 (198.538, -40.2) -> (198.538, -37.251)
  line L1521 (198.538, -37.251) -> (197.7379, -37.251)
  line L1522 (197.7379, -37.251) -> (197.7379, -36.2511)
  line L1523 (197.7379, -36.2511) -> (183.8881, -36.2511)
  line L1524 (202.9381, -36.2511) -> (202.9381, -37.251)
  line L1525 (202.9381, -37.251) -> (202.138, -37.251)
  line L1526 (202.138, -37.251) -> (202.138, -40.2)
  line L1527 (202.138, -40.2) -> (202.9381, -40.2)
  line L1528 (202.9381, -40.2) -> (202.9381, -46.151)
  line L1529 (202.9381, -46.151) -> (202.138, -46.151)
  line L1530 (202.138, -46.151) -> (202.138, -49.1001)
  line L1531 (202.138, -49.1001) -> (202.9381, -49.1001)
  line L1532 (202.9381, -49.1001) -> (202.9381, -50.0999)
  line L1533 (202.9381, -50.0999) -> (216.7879, -50.0999)
  line L1534 (216.7879, -50.0999) -> (216.7879, -49.1001)
  line L1535 (216.7879, -49.1001) -> (217.588, -49.1001)
  line L1536 (217.588, -49.1001) -> (217.588, -46.151)
  line L1537 (217.588, -46.151) -> (216.7879, -46.151)
  line L1538 (216.7879, -46.151) -> (216.7879, -40.2)
  line L1539 (216.7879, -40.2) -> (217.588, -40.2)
  line L1540 (217.588, -40.2) -> (217.588, -37.251)
  line L1541 (217.588, -37.251) -> (216.7879, -37.251)
  line L1542 (216.7879, -37.251) -> (216.7879, -36.2511)
  line L1543 (216.7879, -36.2511) -> (202.9381, -36.2511)
  line L1544 (221.9881, -36.2511) -> (221.9881, -37.251)
  line L1545 (221.9881, -37.251) -> (221.188, -37.251)
  line L1546 (221.188, -37.251) -> (221.188, -40.2)
  line L1547 (221.188, -40.2) -> (221.9881, -40.2)
  line L1548 (221.9881, -40.2) -> (221.9881, -46.151)
  line L1549 (221.9881, -46.151) -> (221.188, -46.151)
  line L1550 (221.188, -46.151) -> (221.188, -49.1001)
  line L1551 (221.188, -49.1001) -> (221.9881, -49.1001)
  line L1552 (221.9881, -49.1001) -> (221.9881, -50.0999)
  line L1553 (221.9881, -50.0999) -> (235.8379, -50.0999)
  line L1554 (235.8379, -50.0999) -> (235.8379, -49.1001)
  line L1555 (235.8379, -49.1001) -> (236.638, -49.1001)
  line L1556 (236.638, -49.1001) -> (236.638, -46.151)
  line L1557 (236.638, -46.151) -> (235.8379, -46.151)
  line L1558 (235.8379, -46.151) -> (235.8379, -40.2)
  line L1559 (235.8379, -40.2) -> (236.638, -40.2)
  line L1560 (236.638, -40.2) -> (236.638, -37.251)
  line L1561 (236.638, -37.251) -> (235.8379, -37.251)
  line L1562 (235.8379, -37.251) -> (235.8379, -36.2511)
  line L1563 (235.8379, -36.2511) -> (221.9881, -36.2511)
  line L1564 (241.0381, -36.2511) -> (241.0381, -37.251)
  line L1565 (241.0381, -37.251) -> (240.238, -37.251)
  line L1566 (240.238, -37.251) -> (240.238, -40.2)
  line L1567 (240.238, -40.2) -> (241.0381, -40.2)
  line L1568 (241.0381, -40.2) -> (241.0381, -46.151)
  line L1569 (241.0381, -46.151) -> (240.238, -46.151)
  line L1570 (240.238, -46.151) -> (240.238, -49.1001)
  line L1571 (240.238, -49.1001) -> (241.0381, -49.1001)
  line L1572 (241.0381, -49.1001) -> (241.0381, -50.0999)
  line L1573 (241.0381, -50.0999) -> (254.8879, -50.0999)
  line L1574 (254.8879, -50.0999) -> (254.8879, -49.1001)
  line L1575 (254.8879, -49.1001) -> (255.688, -49.1001)
  line L1576 (255.688, -49.1001) -> (255.688, -46.151)
  line L1577 (255.688, -46.151) -> (254.8879, -46.151)
  line L1578 (254.8879, -46.151) -> (254.8879, -40.2)
  line L1579 (254.8879, -40.2) -> (255.688, -40.2)
  line L1580 (255.688, -40.2) -> (255.688, -37.251)
  line L1581 (255.688, -37.251) -> (254.8879, -37.251)
  line L1582 (254.8879, -37.251) -> (254.8879, -36.2511)
  line L1583 (254.8879, -36.2511) -> (241.0381, -36.2511)
  line L1584 (12.438, -12.438) -> (12.438, -13.438)
  line L1585 (12.438, -13.438) -> (11.638, -13.438)
  line L1586 (11.638, -13.438) -> (11.638, -16.388)
  line L1587 (11.638, -16.388) -> (12.438, -16.388)
  line L1588 (12.438, -16.388) -> (12.438, -22.338)
  line L1589 (12.438, -22.338) -> (11.638, -22.338)
  line L1590 (11.638, -22.338) -> (11.638, -25.288)
  line L1591 (11.638, -25.288) -> (12.438, -25.288)
  line L1592 (12.438, -25.288) -> (12.438, -26.288)
  line L1593 (12.438, -26.288) -> (26.288, -26.288)
  line L1594 (26.288, -26.288) -> (26.288, -25.288)
  line L1595 (26.288, -25.288) -> (27.088, -25.288)
  line L1596 (27.088, -25.288) -> (27.088, -22.338)
  line L1597 (27.088, -22.338) -> (26.288, -22.338)
  line L1598 (26.288, -22.338) -> (26.288, -16.388)
  line L1599 (26.288, -16.388) -> (27.088, -16.388)
  line L1600 (27.088, -16.388) -> (27.088, -13.438)
  line L1601 (27.088, -13.438) -> (26.288, -13.438)
  line L1602 (26.288, -13.438) -> (26.288, -12.438)
  line L1603 (26.288, -12.438) -> (12.438, -12.438)
  line L1604 (36.2511, -12.438) -> (36.2511, -13.438)
  line L1605 (36.2511, -13.438) -> (35.4499, -13.438)
  line L1606 (35.4499, -13.438) -> (35.4499, -16.388)
  line L1607 (35.4499, -16.388) -> (36.2511, -16.388)
  line L1608 (36.2511, -16.388) -> (36.2511, -22.338)
  line L1609 (36.2511, -22.338) -> (35.4499, -22.338)
  line L1610 (35.4499, -22.338) -> (35.4499, -25.288)
  line L1611 (35.4499, -25.288) -> (36.2511, -25.288)
  line L1612 (36.2511, -25.288) -> (36.2511, -26.288)
  line L1613 (36.2511, -26.288) -> (50.0999, -26.288)
  line L1614 (50.0999, -26.288) -> (50.0999, -25.288)
  line L1615 (50.0999, -25.288) -> (50.9011, -25.288)
  line L1616 (50.9011, -25.288) -> (50.9011, -22.338)
  line L1617 (50.9011, -22.338) -> (50.0999, -22.338)
  line L1618 (50.0999, -22.338) -> (50.0999, -16.388)
  line L1619 (50.0999, -16.388) -> (50.9011, -16.388)
  line L1620 (50.9011, -16.388) -> (50.9011, -13.438)
  line L1621 (50.9011, -13.438) -> (50.0999, -13.438)
  line L1622 (50.0999, -13.438) -> (50.0999, -12.438)
  line L1623 (50.0999, -12.438) -> (36.2511, -12.438)
  line L1624 (55.3011, -12.438) -> (55.3011, -13.438)
  line L1625 (55.3011, -13.438) -> (54.4999, -13.438)
  line L1626 (54.4999, -13.438) -> (54.4999, -16.388)
  line L1627 (54.4999, -16.388) -> (55.3011, -16.388)
  line L1628 (55.3011, -16.388) -> (55.3011, -22.338)
  line L1629 (55.3011, -22.338) -> (54.4999, -22.338)
  line L1630 (54.4999, -22.338) -> (54.4999, -25.288)
  line L1631 (54.4999, -25.288) -> (55.3011, -25.288)
  line L1632 (55.3011, -25.288) -> (55.3011, -26.288)
  line L1633 (55.3011, -26.288) -> (69.1499, -26.288)
  line L1634 (69.1499, -26.288) -> (69.1499, -25.288)
  line L1635 (69.1499, -25.288) -> (69.95, -25.288)
  line L1636 (69.95, -25.288) -> (69.95, -22.338)
  line L1637 (69.95, -22.338) -> (69.1499, -22.338)
  line L1638 (69.1499, -22.338) -> (69.1499, -16.388)
  line L1639 (69.1499, -16.388) -> (69.95, -16.388)
  line L1640 (69.95, -16.388) -> (69.95, -13.438)
  line L1641 (69.95, -13.438) -> (69.1499, -13.438)
  line L1642 (69.1499, -13.438) -> (69.1499, -12.438)
  line L1643 (69.1499, -12.438) -> (55.3011, -12.438)
  line L1644 (74.3511, -12.438) -> (74.3511, -13.438)
  line L1645 (74.3511, -13.438) -> (73.551, -13.438)
  line L1646 (73.551, -13.438) -> (73.551, -16.388)
  line L1647 (73.551, -16.388) -> (74.3511, -16.388)
  line L1648 (74.3511, -16.388) -> (74.3511, -22.338)
  line L1649 (74.3511, -22.338) -> (73.551, -22.338)
  line L1650 (73.551, -22.338) -> (73.551, -25.288)
  line L1651 (73.551, -25.288) -> (74.3511, -25.288)
  line L1652 (74.3511, -25.288) -> (74.3511, -26.288)
  line L1653 (74.3511, -26.288) -> (88.1999, -26.288)
  line L1654 (88.1999, -26.288) -> (88.1999, -25.288)
  line L1655 (88.1999, -25.288) -> (89, -25.288)
  line L1656 (89, -25.288) -> (89, -22.338)
  line L1657 (89, -22.338) -> (88.1999, -22.338)
  line L1658 (88.1999, -22.338) -> (88.1999, -16.388)
  line L1659 (88.1999, -16.388) -> (89, -16.388)
  line L1660 (89, -16.388) -> (89, -13.438)
  line L1661 (89, -13.438) -> (88.1999, -13.438)
  line L1662 (88.1999, -13.438) -> (88.1999, -12.438)
  line L1663 (88.1999, -12.438) -> (74.3511, -12.438)
  line L1664 (93.4, -12.438) -> (93.4, -13.438)
  line L1665 (93.4, -13.438) -> (92.601, -13.438)
  line L1666 (92.601, -13.438) -> (92.601, -16.388)
  line L1667 (92.601, -16.388) -> (93.4, -16.388)
  line L1668 (93.4, -16.388) -> (93.4, -22.338)
  line L1669 (93.4, -22.338) -> (92.601, -22.338)
  line L1670 (92.601, -22.338) -> (92.601, -25.288)
  line L1671 (92.601, -25.288) -> (93.4, -25.288)
  line L1672 (93.4, -25.288) -> (93.4, -26.288)
  line L1673 (93.4, -26.288) -> (107.2499, -26.288)
  line L1674 (107.2499, -26.288) -> (107.2499, -25.288)
  line L1675 (107.2499, -25.288) -> (108.05, -25.288)
  line L1676 (108.05, -25.288) -> (108.05, -22.338)
  line L1677 (108.05, -22.338) -> (107.2499, -22.338)
  line L1678 (107.2499, -22.338) -> (107.2499, -16.388)
  line L1679 (107.2499, -16.388) -> (108.05, -16.388)
  line L1680 (108.05, -16.388) -> (108.05, -13.438)
  line L1681 (108.05, -13.438) -> (107.2499, -13.438)
  line L1682 (107.2499, -13.438) -> (107.2499, -12.438)
  line L1683 (107.2499, -12.438) -> (93.4, -12.438)
  line L1684 (117.2131, -12.438) -> (117.2131, -13.438)
  line L1685 (117.2131, -13.438) -> (116.413, -13.438)
  line L1686 (116.413, -13.438) -> (116.413, -16.388)
  line L1687 (116.413, -16.388) -> (117.2131, -16.388)
  line L1688 (117.2131, -16.388) -> (117.2131, -22.338)
  line L1689 (117.2131, -22.338) -> (116.413, -22.338)
  line L1690 (116.413, -22.338) -> (116.413, -25.288)
  line L1691 (116.413, -25.288) -> (117.2131, -25.288)
  line L1692 (117.2131, -25.288) -> (117.2131, -26.288)
  line L1693 (117.2131, -26.288) -> (131.0629, -26.288)
  line L1694 (131.0629, -26.288) -> (131.0629, -25.288)
  line L1695 (131.0629, -25.288) -> (131.863, -25.288)
  line L1696 (131.863, -25.288) -> (131.863, -22.338)
  line L1697 (131.863, -22.338) -> (131.0629, -22.338)
  line L1698 (131.0629, -22.338) -> (131.0629, -16.388)
  line L1699 (131.0629, -16.388) -> (131.863, -16.388)
  line L1700 (131.863, -16.388) -> (131.863, -13.438)
  line L1701 (131.863, -13.438) -> (131.0629, -13.438)
  line L1702 (131.0629, -13.438) -> (131.0629, -12.438)
  line L1703 (131.0629, -12.438) -> (117.2131, -12.438)
  line L1704 (136.2631, -12.438) -> (136.2631, -13.438)
  line L1705 (136.2631, -13.438) -> (135.463, -13.438)
  line L1706 (135.463, -13.438) -> (135.463, -16.388)
  line L1707 (135.463, -16.388) -> (136.2631, -16.388)
  line L1708 (136.2631, -16.388) -> (136.2631, -22.338)
  line L1709 (136.2631, -22.338) -> (135.463, -22.338)
  line L1710 (135.463, -22.338) -> (135.463, -25.288)
  line L1711 (135.463, -25.288) -> (136.2631, -25.288)
  line L1712 (136.2631, -25.288) -> (136.2631, -26.288)
  line L1713 (136.2631, -26.288) -> (150.1129, -26.288)
  line L1714 (150.1129, -26.288) -> (150.1129, -25.288)
  line L1715 (150.1129, -25.288) -> (150.913, -25.288)
  line L1716 (150.913, -25.288) -> (150.913, -22.338)
  line L1717 (150.913, -22.338) -> (150.1129, -22.338)
  line L1718 (150.1129, -22.338) -> (150.1129, -16.388)
  line L1719 (150.1129, -16.388) -> (150.913, -16.388)
  line L1720 (150.913, -16.388) -> (150.913, -13.438)
  line L1721 (150.913, -13.438) -> (150.1129, -13.438)
  line L1722 (150.1129, -13.438) -> (150.1129, -12.438)
  line L1723 (150.1129, -12.438) -> (136.2631, -12.438)
  line L1724 (155.3131, -12.438) -> (155.3131, -13.438)
  line L1725 (155.3131, -13.438) -> (154.513, -13.438)
  line L1726 (154.513, -13.438) -> (154.513, -16.388)
  line L1727 (154.513, -16.388) -> (155.3131, -16.388)
  line L1728 (155.3131, -16.388) -> (155.3131, -22.338)
  line L1729 (155.3131, -22.338) -> (154.513, -22.338)
  line L1730 (154.513, -22.338) -> (154.513, -25.288)
  line L1731 (154.513, -25.288) -> (155.3131, -25.288)
  line L1732 (155.3131, -25.288) -> (155.3131, -26.288)
  line L1733 (155.3131, -26.288) -> (169.1629, -26.288)
  line L1734 (169.1629, -26.288) -> (169.1629, -25.288)
  line L1735 (169.1629, -25.288) -> (169.963, -25.288)
  line L1736 (169.963, -25.288) -> (169.963, -22.338)
  line L1737 (169.963, -22.338) -> (169.1629, -22.338)
  line L1738 (169.1629, -22.338) -> (169.1629, -16.388)
  line L1739 (169.1629, -16.388) -> (169.963, -16.388)
  line L1740 (169.963, -16.388) -> (169.963, -13.438)
  line L1741 (169.963, -13.438) -> (169.1629, -13.438)
  line L1742 (169.1629, -13.438) -> (169.1629, -12.438)
  line L1743 (169.1629, -12.438) -> (155.3131, -12.438)
  line L1744 (174.3631, -12.438) -> (174.3631, -13.438)
  line L1745 (174.3631, -13.438) -> (173.563, -13.438)
  line L1746 (173.563, -13.438) -> (173.563, -16.388)
  line L1747 (173.563, -16.388) -> (174.3631, -16.388)
  line L1748 (174.3631, -16.388) -> (174.3631, -22.338)
  line L1749 (174.3631, -22.338) -> (173.563, -22.338)
  line L1750 (173.563, -22.338) -> (173.563, -25.288)
  line L1751 (173.563, -25.288) -> (174.3631, -25.288)
  line L1752 (174.3631, -25.288) -> (174.3631, -26.288)
  line L1753 (174.3631, -26.288) -> (188.2129, -26.288)
  line L1754 (188.2129, -26.288) -> (188.2129, -25.288)
  line L1755 (188.2129, -25.288) -> (189.013, -25.288)
  line L1756 (189.013, -25.288) -> (189.013, -22.338)
  line L1757 (189.013, -22.338) -> (188.2129, -22.338)
  line L1758 (188.2129, -22.338) -> (188.2129, -16.388)
  line L1759 (188.2129, -16.388) -> (189.013, -16.388)
  line L1760 (189.013, -16.388) -> (189.013, -13.438)
  line L1761 (189.013, -13.438) -> (188.2129, -13.438)
  line L1762 (188.2129, -13.438) -> (188.2129, -12.438)
  line L1763 (188.2129, -12.438) -> (174.3631, -12.438)
  line L1764 (198.1761, -12.438) -> (198.1761, -13.438)
  line L1765 (198.1761, -13.438) -> (197.376, -13.438)
  line L1766 (197.376, -13.438) -> (197.376, -16.388)
  line L1767 (197.376, -16.388) -> (198.1761, -16.388)
  line L1768 (198.1761, -16.388) -> (198.1761, -22.338)
  line L1769 (198.1761, -22.338) -> (197.376, -22.338)
  line L1770 (197.376, -22.338) -> (197.376, -25.288)
  line L1771 (197.376, -25.288) -> (198.1761, -25.288)
  line L1772 (198.1761, -25.288) -> (198.1761, -26.288)
  line L1773 (198.1761, -26.288) -> (212.026, -26.288)
  line L1774 (212.026, -26.288) -> (212.026, -25.288)
  line L1775 (212.026, -25.288) -> (212.8261, -25.288)
  line L1776 (212.8261, -25.288) -> (212.8261, -22.338)
  line L1777 (212.8261, -22.338) -> (212.026, -22.338)
  line L1778 (212.026, -22.338) -> (212.026, -16.388)
  line L1779 (212.026, -16.388) -> (212.8261, -16.388)
  line L1780 (212.8261, -16.388) -> (212.8261, -13.438)
  line L1781 (212.8261, -13.438) -> (212.026, -13.438)
  line L1782 (212.026, -13.438) -> (212.026, -12.438)
  line L1783 (212.026, -12.438) -> (198.1761, -12.438)
  line L1784 (217.2261, -12.438) -> (217.2261, -13.438)
  line L1785 (217.2261, -13.438) -> (216.426, -13.438)
  line L1786 (216.426, -13.438) -> (216.426, -16.388)
  line L1787 (216.426, -16.388) -> (217.2261, -16.388)
  line L1788 (217.2261, -16.388) -> (217.2261, -22.338)
  line L1789 (217.2261, -22.338) -> (216.426, -22.338)
  line L1790 (216.426, -22.338) -> (216.426, -25.288)
  line L1791 (216.426, -25.288) -> (217.2261, -25.288)
  line L1792 (217.2261, -25.288) -> (217.2261, -26.288)
  line L1793 (217.2261, -26.288) -> (231.076, -26.288)
  line L1794 (231.076, -26.288) -> (231.076, -25.288)
  line L1795 (231.076, -25.288) -> (231.8761, -25.288)
  line L1796 (231.8761, -25.288) -> (231.8761, -22.338)
  line L1797 (231.8761, -22.338) -> (231.076, -22.338)
  line L1798 (231.076, -22.338) -> (231.076, -16.388)
  line L1799 (231.076, -16.388) -> (231.8761, -16.388)
  line L1800 (231.8761, -16.388) -> (231.8761, -13.438)
  line L1801 (231.8761, -13.438) -> (231.076, -13.438)
  line L1802 (231.076, -13.438) -> (231.076, -12.438)
  line L1803 (231.076, -12.438) -> (217.2261, -12.438)
  line L1804 (236.2761, -12.438) -> (236.2761, -13.438)
  line L1805 (236.2761, -13.438) -> (235.476, -13.438)
  line L1806 (235.476, -13.438) -> (235.476, -16.388)
  line L1807 (235.476, -16.388) -> (236.2761, -16.388)